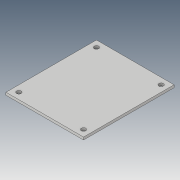
# Autodesk Inventor part: Supporto1
Saved by Autodesk Inventor 2019 (Build 230136000, 136)
## iProperties
Created: 2019-07-23
Part Number: Supporto1
Material: Generic
Document SubType Name: Modeling
Designer: giacomo
Density: 1 g/cm^3
Appearance: Default
Author: giacomo
Autodesk Inventor part; units mm, degrees
ref_plane "YZ Plane" through (0, 0, 0) normal (1, 0, 0) x (0, 1, 0)
ref_plane "XZ Plane" through (0, 0, 0) normal (0, 1, 0) x (-1, 0, 0)
ref_plane "XY Plane" through (0, 0, 0) normal (0, 0, 1) x (1, 0, 0)
sketch "Sketch1" plane through (0, 0, 0) normal (0, 1, 0) x (-1, 0, 0)
  line L0 (30, 48.6275) -> (-30, 48.6275)
  line L1 (-30, 48.6275) -> (-30, -21.3725)
  line L2 (-30, -21.3725) -> (30, -21.3725)
  line L3 (30, -21.3725) -> (30, 48.6275)
  point P0 (0, 0)
  dimension "d0" = 70
  dimension "d1" = 60
  constraints: 8 end point, 2 parallel, 1 horizontal, 1 perpendicular
  measures "d0" distance of L2.end L0.start
  measures "d1" distance of L0.start L0.end
extrude "Extrusion1" add sketch "Sketch1" along normal blind 2
sketch "Sketch2" plane through (0, 2, 0) normal (0, 1, 0) x (1, 0, 0)
  line L0 (0, 0) -> (-21.5262, 0) construction
  circle A0 centre (-25, -43.6275) radius 1.75
  line L1 (-30, -48.6275) -> (30, -48.6275) projected
  line L2 (-30, 21.3725) -> (-30, -48.6275) projected
  circle A1 centre (25, -43.6275) radius 1.75
  circle A2 centre (25, 16.3725) radius 1.75
  circle A3 centre (-25, 16.3725) radius 1.75
  line L3 (30, -48.6275) -> (30, 21.3725) projected
  line L4 (30, 21.3725) -> (-30, 21.3725) projected
  dimension "d4" = 3.5
  dimension "d5" = 5
  dimension "d6" = 5
  dimension "d7" = 3.5
  dimension "d8" = 3.5
  dimension "d9" = 3.5
  dimension "d10" = 5
  dimension "d11" = 5
  dimension "d12" = 5
  dimension "d13" = 5
  dimension "d14" = 5
  dimension "d15" = 5
  constraints: 4 centre point, 2 end point, 1 horizontal
  measures "d4" diameter of A0
  measures "d5" distance from line of L1 A0.centre
  measures "d6" distance from line of L2 A0.centre
  measures "d7" diameter of A1
  measures "d8" diameter of A2
  measures "d9" diameter of A3
  measures "d10" distance from line of L3 A1.centre
  measures "d11" distance from line of L1 A1.centre
  measures "d12" distance from line of L2 A3.centre
  measures "d13" distance from line of L4 A3.centre
  measures "d14" distance from line of L3 A2.centre
  measures "d15" distance from line of L4 A2.centre
extrude "Extrusion2" cut sketch "Sketch2" against normal through all contours A0 | A1 | A2 | A3
body "Solid1"
